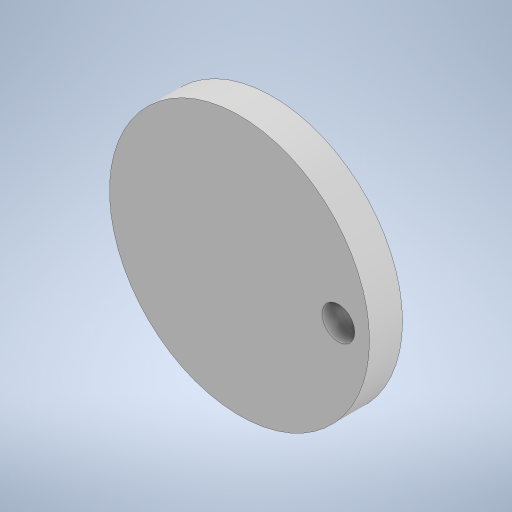
# Autodesk Inventor part: Wheel_Consept
Saved by Autodesk Inventor 2024 (Build 280153000, 153)
## iProperties
Created: 2024-01-13
Part Number: Wheel_Consept
Material: Generic
Document SubType Name: Modeling
Designer: Owner
Density: 1 g/cm^3
Appearance: Default
Author: Owner
Autodesk Inventor part; units mm, degrees
ref_plane "YZ Plane" through (0, 0, 0) normal (1, 0, 0) x (0, 1, 0)
ref_plane "XZ Plane" through (0, 0, 0) normal (0, 1, 0) x (-1, 0, 0)
ref_plane "XY Plane" through (0, 0, 0) normal (0, 0, 1) x (1, 0, 0)
sketch "Sketch1" plane through (0, 0, 0) normal (0, 0, 1) x (1, 0, 0)
  circle A0 centre (0, 0) radius 500
  dimension "d0" = 1000
  constraints: 1 centre point, 1 coincident
  measures "d0" diameter of A0
extrude "Extrusion1" add sketch "Sketch1" along normal blind 127
sketch "Sketch3" plane through (0, 0, 127) normal (0, 0, 1) x (1, 0, 0)
  circle A0 centre (380.6947, -1.1254) radius 62.8623
  point P0 (0, 0)
  dimension "d3" = 125.7246
  dimension "d4" = 380.6964
  constraints: 1 centre point
  measures "d3" diameter of A0
  measures "d4" distance of A0.centre point (0, 0)
extrude "Extrusion2" cut sketch "Sketch3" against normal blind 127
body "Solid1"
